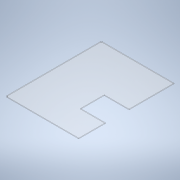
# Autodesk Inventor part: MountingWallSide
Saved by Autodesk Inventor 2020 (Build 240168000, 168)
## iProperties
Created: 2020-04-26
Part Number: MountingWallSide
Material: Типовые
Document SubType Name: Modeling
Designer: Михаил
Density: 1 g/cm^3
Appearance: По умолчанию
Author: Михаил
Autodesk Inventor part; units mm, degrees
ref_plane "YZ Plane" through (0, 0, 0) normal (1, 0, 0) x (0, 1, 0)
ref_plane "XZ Plane" through (0, 0, 0) normal (0, 1, 0) x (-1, 0, 0)
ref_plane "XY Plane" through (0, 0, 0) normal (0, 0, 1) x (1, 0, 0)
sketch "Эскиз1" plane through (0, 0, 0) normal (0, 1, 0) x (-1, 0, 0)
  line L0 (0, 0) -> (388, 0)
  line L1 (388, 0) -> (388, -508)
  line L2 (388, -508) -> (0, -508)
  line L3 (0, -508) -> (0, 0)
  dimension "d0" = 388
  dimension "d1" = 508
  constraints: 8 end point, 2 parallel, 1 horizontal, 1 perpendicular
  measures "d0" distance of L1.end L2.end
  measures "d1" distance of L0.end L1.end
extrude "Выдавливание1" add sketch "Эскиз1" along normal blind 4
sketch "Эскиз2" plane through (0, 4, 0) normal (0, 1, 0) x (1, 0, 0)
  line L0 (0, 0) -> (0, 508) projected
  line L1 (0, 142) -> (-132, 142)
  line L2 (-132, 142) -> (-132, 268)
  line L3 (-132, 268) -> (0, 268)
  line L4 (0, 268) -> (0, 142)
  line L5 (-388, 0) -> (0, 0) projected
  point P0 (0, 268)
  dimension "d4" = 132
  dimension "d5" = 126
  dimension "d6" = 142
  constraints: 8 end point, 2 parallel, 1 horizontal, 1 perpendicular, 1 point on line
  measures "d4" distance of L2.end L3.end
  measures "d5" distance of L1.end L2.end
  measures "d6" distance between parallel lines of L1 L5
extrude "Выдавливание2" cut sketch "Эскиз2" against normal blind 4
sketch "Эскиз3" plane through (0, 4, 0) normal (0, 1, 0) x (1, 0, 0)
  line L0 (-388, 0) -> (0, 0) projected
  line L1 (-388, 0) -> (-384, 0)
  line L2 (-384, 0) -> (-384, 4)
  line L3 (-384, 4) -> (-388, 4)
  line L4 (-388, 4) -> (-388, 0)
  line L5 (-388, 508) -> (-388, 0) projected
  line L6 (-388, 508) -> (-384, 508)
  line L7 (-384, 508) -> (-384, 504)
  line L8 (-384, 504) -> (-388, 504)
  line L9 (-388, 504) -> (-388, 508)
  dimension "d9" = 4
  dimension "d10" = 4
  dimension "d11" = 4
  dimension "d12" = 4
  constraints: 16 end point, 4 parallel, 2 horizontal, 2 perpendicular
  measures "d9" distance of L3.end L2.end
  measures "d10" distance of L2.end L1.end
  measures "d11" distance of L7.end L8.end
  measures "d12" distance of L6.end L7.end
extrude "Выдавливание3" cut sketch "Эскиз3" against normal blind 4
